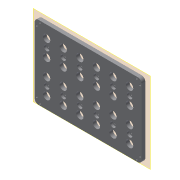
# Autodesk Inventor part: 06_Omniscope_lid_lenses
Saved by Autodesk Inventor 2019 (Build 230136000, 136)
## iProperties
Created: 2021-09-23
Part Number: 06_Omniscope_lid_lenses
Material: Generisch
Document SubType Name: Modeling
Designer: Muriel
Density: 1 g/cm^3
Appearance: Vorgabe
Author: Muriel
Autodesk Inventor part; units mm, degrees
ref_plane "YZ Plane" through (0, 0, 0) normal (1, 0, 0) x (0, 1, 0)
ref_plane "XZ Plane" through (0, 0, 0) normal (0, 1, 0) x (-1, 0, 0)
ref_plane "XY Plane" through (0, 0, 0) normal (0, 0, 1) x (1, 0, 0)
ref_plane "Arbeitsebene1" through (0, 0, 0) normal (0, 0, 1) x (1, 0, 0)
sketch "Skizze1" plane through (0, 0, 0) normal (0, 0, 1) x (1, 0, 0)
  circle A0 centre (-56, 33.5) radius 0.9 projected
  circle A1 centre (-52.5, -38) radius 0.9 projected
  circle A2 centre (56, -33.5) radius 0.9 projected
  circle A3 centre (52.5, 38) radius 0.9 projected
  circle A4 centre (56, 33.5) radius 0.9 projected
  circle A5 centre (52.5, -38) radius 0.9 projected
  circle A6 centre (-56, -33.5) radius 0.9 projected
  circle A7 centre (-52.5, 38) radius 0.9 projected
  line L0 (54.4717, 36.4176) -> (-54.4717, 36.4176) projected
  line L1 (54.4717, -36.4176) -> (54.4717, 36.4176) projected
  line L2 (-54.4717, -36.4176) -> (54.4717, -36.4176) projected
  line L3 (-54.4717, 36.4176) -> (-54.4717, -36.4176) projected
  arc A8 (-57.9717, -35.9176) -> (-53.9717, -39.9176) centre (-53.9717, -35.9176) ccw projected
  line L4 (53.9717, -39.9176) -> (-53.9717, -39.9176) projected
  arc A9 (53.9717, -39.9176) -> (57.9717, -35.9176) centre (53.9717, -35.9176) ccw projected
  line L5 (57.9717, 35.9176) -> (57.9717, -35.9176) projected
  arc A10 (57.9717, 35.9176) -> (53.9717, 39.9176) centre (53.9717, 35.9176) ccw projected
  line L6 (-53.9717, 39.9176) -> (53.9717, 39.9176) projected
  arc A11 (-53.9717, 39.9176) -> (-57.9717, 35.9176) centre (-53.9717, 35.9176) ccw projected
  line L7 (-57.9717, -35.9176) -> (-57.9717, 35.9176) projected
  circle A12 centre (44.9634, -18.0176) radius 1.4 projected
  circle A13 centre (26.9634, -18.0176) radius 1.4 projected
  circle A14 centre (8.9634, -18.0176) radius 1.4 projected
  circle A15 centre (-9.0366, -18.0176) radius 1.4 projected
  circle A16 centre (-27.0366, -18.0176) radius 1.4 projected
  circle A17 centre (-45.0366, -18.0176) radius 1.4 projected
  circle A18 centre (-45.0366, 17.9824) radius 1.4 projected
  circle A19 centre (-27.0366, 17.9824) radius 1.4 projected
  circle A20 centre (-9.0366, 17.9824) radius 1.4 projected
  circle A21 centre (8.9634, 17.9824) radius 1.4 projected
  circle A22 centre (26.9634, 17.9824) radius 1.4 projected
  circle A23 centre (44.9634, 17.9824) radius 1.4 projected
  circle A24 centre (44.9634, -26.9676) radius 4 projected
  circle A25 centre (26.9634, -26.9676) radius 4 projected
  circle A26 centre (8.9634, -26.9676) radius 4 projected
  circle A27 centre (-9.0366, -26.9676) radius 4 projected
  circle A28 centre (-27.0366, -26.9676) radius 4 projected
  circle A29 centre (-45.0366, -26.9676) radius 4 projected
  circle A30 centre (-45.0366, -9.0676) radius 4 projected
  circle A31 centre (-27.0366, -9.0676) radius 4 projected
  circle A32 centre (-9.0366, -9.0676) radius 4 projected
  circle A33 centre (8.9634, -9.0676) radius 4 projected
  circle A34 centre (26.9634, -9.0676) radius 4 projected
  line L8 (47.4634, -11.0176) -> (47.4634, -8.0176) projected
  circle A35 centre (44.9634, -9.0676) radius 4 projected
  circle A36 centre (44.9634, 9.0324) radius 4 projected
  circle A37 centre (44.9634, 26.9324) radius 4 projected
  circle A38 centre (26.9634, 9.0324) radius 4 projected
  circle A39 centre (26.9634, 26.9324) radius 4 projected
  circle A40 centre (8.9634, 9.0324) radius 4 projected
  circle A41 centre (8.9634, 26.9324) radius 4 projected
  circle A42 centre (-9.0366, 26.9324) radius 4 projected
  circle A43 centre (-9.0366, 9.0324) radius 4 projected
  circle A44 centre (-27.0366, 9.0324) radius 4 projected
  circle A45 centre (-27.0366, 26.9324) radius 4.2 projected
  circle A46 centre (-45.0366, 9.0324) radius 4.2 projected
  circle A47 centre (-45.0366, 26.9324) radius 4 projected
  point P0 (0, 0)
extrude "Extrusion1" add sketch "Skizze1" along normal blind 2 contours L1 L2 L3 L0 | L7 A11 L6 A10 L5 A9 L4 A8
sketch "Skizze2" plane through (0, 0, 2) normal (0, 0, 1) x (1, 0, 0)
  circle A0 centre (-45.0366, 9.0324) radius 4.2 projected
  circle A1 centre (-27.0366, 26.9324) radius 4.2 projected
  circle A2 centre (-45.0366, 26.9324) radius 4 projected
  circle A3 centre (-27.0366, 9.0324) radius 4 projected
  circle A4 centre (-9.0366, 9.0324) radius 4 projected
  circle A5 centre (-9.0366, 26.9324) radius 4 projected
  circle A6 centre (8.9634, 26.9324) radius 4 projected
  circle A7 centre (8.9634, 9.0324) radius 4 projected
  circle A8 centre (26.9634, 26.9324) radius 4 projected
  circle A9 centre (26.9634, 9.0324) radius 4 projected
  circle A10 centre (44.9634, 26.9324) radius 4 projected
  circle A11 centre (44.9634, 9.0324) radius 4 projected
  circle A12 centre (44.9634, -9.0676) radius 4 projected
  circle A13 centre (26.9634, -9.0676) radius 4 projected
  circle A14 centre (8.9634, -9.0676) radius 4 projected
  circle A15 centre (-9.0366, -9.0676) radius 4 projected
  circle A16 centre (-27.0366, -9.0676) radius 4 projected
  circle A17 centre (-45.0366, -9.0676) radius 4 projected
  circle A18 centre (-45.0366, -26.9676) radius 4 projected
  circle A19 centre (-27.0366, -26.9676) radius 4 projected
  circle A20 centre (-9.0366, -26.9676) radius 4 projected
  circle A21 centre (8.9634, -26.9676) radius 4 projected
  circle A22 centre (26.9634, -26.9676) radius 4 projected
  circle A23 centre (44.9634, -26.9676) radius 4 projected
  circle A24 centre (44.9634, 17.9824) radius 1.4 projected
  circle A25 centre (26.9634, 17.9824) radius 1.4 projected
  circle A26 centre (8.9634, 17.9824) radius 1.4 projected
  circle A27 centre (-9.0366, 17.9824) radius 1.4 projected
  circle A28 centre (-27.0366, 17.9824) radius 1.4 projected
  circle A29 centre (-45.0366, 17.9824) radius 1.4 projected
  circle A30 centre (-45.0366, -18.0176) radius 1.4 projected
  circle A31 centre (-27.0366, -18.0176) radius 1.4 projected
  circle A32 centre (-9.0366, -18.0176) radius 1.4 projected
  circle A33 centre (8.9634, -18.0176) radius 1.4 projected
  circle A34 centre (26.9634, -18.0176) radius 1.4 projected
  circle A35 centre (44.9634, -18.0176) radius 1.4 projected
  circle A36 centre (-52.5, 38) radius 0.9 projected
  circle A37 centre (-56, -33.5) radius 0.9 projected
  circle A38 centre (52.5, -38) radius 0.9 projected
  circle A39 centre (56, 33.5) radius 0.9 projected
  circle A40 centre (52.5, 38) radius 0.9 projected
  circle A41 centre (56, -33.5) radius 0.9 projected
  circle A42 centre (-52.5, -38) radius 0.9 projected
  circle A43 centre (-56, 33.5) radius 0.9 projected
  arc A44 (-57.9717, -35.9176) -> (-53.9717, -39.9176) centre (-53.9717, -35.9176) ccw projected
  line L0 (-53.9717, -39.9176) -> (53.9717, -39.9176) projected
  arc A45 (53.9717, -39.9176) -> (57.9717, -35.9176) centre (53.9717, -35.9176) ccw projected
  line L1 (57.9717, -35.9176) -> (57.9717, 35.9176) projected
  arc A46 (57.9717, 35.9176) -> (53.9717, 39.9176) centre (53.9717, 35.9176) ccw projected
  line L2 (53.9717, 39.9176) -> (-53.9717, 39.9176) projected
  arc A47 (-53.9717, 39.9176) -> (-57.9717, 35.9176) centre (-53.9717, 35.9176) ccw projected
  line L3 (-57.9717, 35.9176) -> (-57.9717, -35.9176) projected
  point P0 (0, 0)
extrude "Extrusion2" add sketch "Skizze2" along normal blind 2 contours A0 | A1 | A2 | A3 | A4 | A5 | A6 | A7 | A8 | A9 | A10 | A11 | A12 | A13 | A14 | A15 | A16 | A17 | A18 | A19 | A20 | A21 | A22 | A23 | L3 A47 L2 A46 L1 A45 L0 A44
sketch "Skizze3" plane through (0, 0, 4) normal (0, 0, 1) x (1, 0, 0)
  circle A0 centre (44.9634, 17.9824) radius 1.4 projected
  circle A1 centre (48.8634, 17.9824) radius 0.1 projected
  line L0 (52.8634, 35.8824) -> (53.8634, 34.8824) projected
  line L1 (37.0634, 35.8824) -> (52.8634, 35.8824) projected
  line L2 (36.0634, 34.8824) -> (37.0634, 35.8824) projected
  line L3 (36.0634, 1.0824) -> (36.0634, 34.8824) projected
  line L4 (37.0634, 0.0824) -> (36.0634, 1.0824) projected
  line L5 (37.0634, 0.0824) -> (52.8634, 0.0824) projected
  line L6 (53.8634, 1.0824) -> (52.8634, 0.0824) projected
  line L7 (53.8634, 1.0824) -> (53.8634, 34.8824) projected
  circle A2 centre (44.9634, 26.9324) radius 4.2 projected
  circle A3 centre (44.9634, 9.0324) radius 4.2 projected
  circle A4 centre (44.9634, 26.9324) radius 3.95
  circle A5 centre (44.9634, 9.0324) radius 3.95
  point P0 (0, 0)
  dimension "d4" = 7.9
  dimension "d7" = 7.9
  constraints: 2 centre point, 2 coincident
  measures "d4" diameter of A4
  measures "d7" diameter of A5
extrude "Extrusion3" cut sketch "Skizze3" against normal blind 2 contours A4 | A5
sketch "Skizze4" plane through (0, 0, 4) normal (0, 0, 1) x (1, 0, 0)
  circle A0 centre (44.9634, 26.9324) radius 3.95 projected
  circle A1 centre (44.9634, 9.0324) radius 3.95 projected
  circle A2 centre (44.9634, -18.0176) radius 1.4 projected
  circle A3 centre (26.9634, -18.0176) radius 1.4 projected
  circle A4 centre (8.9634, -18.0176) radius 1.4 projected
  circle A5 centre (-9.0366, -18.0176) radius 1.4 projected
  circle A6 centre (-27.0366, -18.0176) radius 1.4 projected
  circle A7 centre (-45.0366, -18.0176) radius 1.4 projected
  circle A8 centre (-45.0366, 17.9824) radius 1.4 projected
  circle A9 centre (-27.0366, 17.9824) radius 1.4 projected
  circle A10 centre (-9.0366, 17.9824) radius 1.4 projected
  circle A11 centre (8.9634, 17.9824) radius 1.4 projected
  circle A12 centre (26.9634, 17.9824) radius 1.4 projected
  circle A13 centre (44.9634, 17.9824) radius 1.4 projected
  circle A14 centre (-56, 33.5) radius 0.9 projected
  circle A15 centre (-52.5, -38) radius 0.9 projected
  circle A16 centre (56, -33.5) radius 0.9 projected
  circle A17 centre (52.5, 38) radius 0.9 projected
  circle A18 centre (56, 33.5) radius 0.9 projected
  circle A19 centre (52.5, -38) radius 0.9 projected
  circle A20 centre (-56, -33.5) radius 0.9 projected
  circle A21 centre (-52.5, 38) radius 0.9 projected
  arc A22 (-57.9717, -35.9176) -> (-53.9717, -39.9176) centre (-53.9717, -35.9176) ccw projected
  line L0 (-53.9717, -39.9176) -> (53.9717, -39.9176) projected
  arc A23 (53.9717, -39.9176) -> (57.9717, -35.9176) centre (53.9717, -35.9176) ccw projected
  line L1 (57.9717, -35.9176) -> (57.9717, 35.9176) projected
  arc A24 (57.9717, 35.9176) -> (53.9717, 39.9176) centre (53.9717, 35.9176) ccw projected
  line L2 (53.9717, 39.9176) -> (-53.9717, 39.9176) projected
  arc A25 (-53.9717, 39.9176) -> (-57.9717, 35.9176) centre (-53.9717, 35.9176) ccw projected
  line L3 (-57.9717, 35.9176) -> (-57.9717, -35.9176) projected
  point P0 (0, 0)
hole "Bohrung1" at (44.9634, -18.0176, 4) at (26.9634, -18.0176, 4) at (8.9634, -18.0176, 4) at (-9.0366, -18.0176, 4) at (-27.0366, -18.0176, 4) at (-45.0366, -18.0176, 4) at (-45.0366, 17.9824, 4) at (-27.0366, 17.9824, 4) at (-9.0366, 17.9824, 4) at (8.9634, 17.9824, 4) at (26.9634, 17.9824, 4) at (44.9634, 17.9824, 4) direction (0, 0, -1) diameter 2.8 depth 12 tip angle 118 counterbore diameter 6 counterbore depth 2.5
pattern_linear "Rechteckige Anordnung1" count 2 spacing 36 along (0, -1, 0) count 6 spacing 18 along (-1, 0, 0) of "Extrusion3"
ref_plane "Arbeitsebene2" through (-53.9717, 0, 0) normal (0, 1, 0) x (1, 0, 0)
ref_plane "Arbeitsebene3" through (0, -35.9176, 0) normal (1, 0, 0) x (0, 0, -1)
sketch "Skizze5" plane through (0, 0, 0) normal (0, 0, -1) x (-1, 0, 0)
  circle A0 centre (56, -33.5) radius 0.9 projected
  circle A1 centre (-56, 33.5) radius 0.9 projected
  circle A2 centre (-56, -33.5) radius 0.9 projected
  circle A3 centre (56, 33.5) radius 0.9 projected
  circle A4 centre (52.5, -38) radius 0.9 projected
  circle A5 centre (-52.5, 38) radius 0.9 projected
  circle A6 centre (-52.5, -38) radius 0.9 projected
  circle A7 centre (52.5, 38) radius 0.9 projected
  arc A8 (53.9717, -39.9176) -> (57.9717, -35.9176) centre (53.9717, -35.9176) ccw projected
  line L0 (57.9717, -35.9176) -> (57.9717, 35.9176) projected
  arc A9 (57.9717, 35.9176) -> (53.9717, 39.9176) centre (53.9717, 35.9176) ccw projected
  line L1 (53.9717, 39.9176) -> (-53.9717, 39.9176) projected
  arc A10 (-53.9717, 39.9176) -> (-57.9717, 35.9176) centre (-53.9717, 35.9176) ccw projected
  line L2 (-57.9717, 35.9176) -> (-57.9717, -35.9176) projected
  arc A11 (-57.9717, -35.9176) -> (-53.9717, -39.9176) centre (-53.9717, -35.9176) ccw projected
  line L3 (-53.9717, -39.9176) -> (53.9717, -39.9176) projected
  circle A12 centre (50.0366, -8.0176) radius 1.4 projected
  circle A13 centre (50.0366, -28.0176) radius 1.4 projected
  circle A14 centre (40.0366, -28.0176) radius 1.4 projected
  circle A15 centre (40.0366, -8.0176) radius 1.4 projected
  circle A16 centre (32.0366, -8.0176) radius 1.4 projected
  circle A17 centre (32.0366, -28.0176) radius 1.4 projected
  circle A18 centre (22.0366, -28.0176) radius 1.4 projected
  circle A19 centre (22.0366, -8.0176) radius 1.4 projected
  circle A20 centre (14.0366, -8.0176) radius 1.4 projected
  circle A21 centre (14.0366, -28.0176) radius 1.4 projected
  circle A22 centre (4.0366, -28.0176) radius 1.4 projected
  circle A23 centre (4.0366, -8.0176) radius 1.4 projected
  circle A24 centre (-3.9634, -8.0176) radius 1.4 projected
  circle A25 centre (-3.9634, -28.0176) radius 1.4 projected
  circle A26 centre (-13.9634, -28.0176) radius 1.4 projected
  circle A27 centre (-13.9634, -8.0176) radius 1.4 projected
  circle A28 centre (-21.9634, -8.0176) radius 1.4 projected
  circle A29 centre (-21.9634, -28.0176) radius 1.4 projected
  circle A30 centre (-31.9634, -28.0176) radius 1.4 projected
  circle A31 centre (-31.9634, -8.0176) radius 1.4 projected
  circle A32 centre (-39.9634, -8.0176) radius 1.4 projected
  circle A33 centre (-39.9634, -28.0176) radius 1.4 projected
  circle A34 centre (-49.9634, -28.0176) radius 1.4 projected
  circle A35 centre (-49.9634, -8.0176) radius 1.4 projected
  circle A36 centre (50.0366, 27.9824) radius 1.4 projected
  circle A37 centre (50.0366, 7.9824) radius 1.4 projected
  circle A38 centre (40.0366, 7.9824) radius 1.4 projected
  circle A39 centre (40.0366, 27.9824) radius 1.4 projected
  circle A40 centre (32.0366, 27.9824) radius 1.4 projected
  circle A41 centre (32.0366, 7.9824) radius 1.4 projected
  circle A42 centre (22.0366, 7.9824) radius 1.4 projected
  circle A43 centre (22.0366, 27.9824) radius 1.4 projected
  circle A44 centre (14.0366, 27.9824) radius 1.4 projected
  circle A45 centre (14.0366, 7.9824) radius 1.4 projected
  circle A46 centre (4.0366, 7.9824) radius 1.4 projected
  circle A47 centre (4.0366, 27.9824) radius 1.4 projected
  circle A48 centre (-3.9634, 27.9824) radius 1.4 projected
  circle A49 centre (-3.9634, 7.9824) radius 1.4 projected
  circle A50 centre (-13.9634, 7.9824) radius 1.4 projected
  circle A51 centre (-13.9634, 27.9824) radius 1.4 projected
  circle A52 centre (-21.9634, 27.9824) radius 1.4 projected
  circle A53 centre (-21.9634, 7.9824) radius 1.4 projected
  circle A54 centre (-31.9634, 7.9824) radius 1.4 projected
  circle A55 centre (-31.9634, 27.9824) radius 1.4 projected
  circle A56 centre (-39.9634, 27.9824) radius 1.4 projected
  circle A57 centre (-39.9634, 7.9824) radius 1.4 projected
  circle A58 centre (-49.9634, 7.9824) radius 1.4 projected
  circle A59 centre (-49.9634, 27.9824) radius 1.4 projected
  arc A60 (-61.6851, 35.0492) -> (-61.8, 34.7718) centre (-59.9, 34.1473) ccw projected
  line L4 (-61.8, -34.7718) -> (-61.8, 34.7718) projected
  arc A61 (-61.8, -34.7718) -> (-61.6851, -35.0492) centre (-59.9, -34.1473) ccw projected
  line L5 (-56.1492, -40.5851) -> (-61.6851, -35.0492) projected
  arc A62 (-56.1492, -40.5851) -> (-55.8718, -40.7) centre (-55.2473, -38.8) ccw projected
  line L6 (60.2, -40.7) -> (-55.8718, -40.7) projected
  arc A63 (60.2, -40.7) -> (61.8, -39.1) centre (60.2, -39.1) ccw projected
  line L7 (61.8, 39.1) -> (61.8, -39.1) projected
  arc A64 (61.8, 39.1) -> (60.2, 40.7) centre (60.2, 39.1) ccw projected
  line L8 (-55.8718, 40.7) -> (60.2, 40.7) projected
  arc A65 (-55.8718, 40.7) -> (-56.1492, 40.5851) centre (-55.2473, 38.8) ccw projected
  line L9 (-61.6851, 35.0492) -> (-56.1492, 40.5851) projected
  line L10 (-54.3, 36.3) -> (54.3, 36.3) projected
  line L11 (54.3, 36.3) -> (54.3, -36.3) projected
  line L12 (54.3, -36.3) -> (-54.3, -36.3) projected
  line L13 (-54.3, -36.3) -> (-54.3, 36.3) projected
  arc A66 (-62.3, -34.8473) -> (-62.092, -35.3494) centre (-59.9, -34.1473) ccw
  line L14 (-62.3, -34.8473) -> (-62.3, 34.8473)
  arc A67 (-62.092, 35.3494) -> (-62.3, 34.8473) centre (-59.9, 34.1473) ccw
  line L15 (-62.092, 35.3494) -> (-56.4494, 40.992)
  arc A68 (-55.9473, 41.2) -> (-56.4494, 40.992) centre (-55.2473, 38.8) ccw
  line L16 (-55.9473, 41.2) -> (60.2, 41.2)
  arc A69 (62.3, 39.1) -> (60.2, 41.2) centre (60.2, 39.1) ccw
  line L17 (62.3, 39.1) -> (62.3, -39.1)
  arc A70 (60.2, -41.2) -> (62.3, -39.1) centre (60.2, -39.1) ccw
  line L18 (60.2, -41.2) -> (-55.9473, -41.2)
  arc A71 (-56.4494, -40.992) -> (-55.9473, -41.2) centre (-55.2473, -38.8) ccw
  line L19 (-56.4494, -40.992) -> (-62.092, -35.3494)
  arc A72 (-61.3, -34.6858) -> (-61.2707, -34.7565) centre (-59.9, -34.1473) ccw
  line L20 (-61.3, -34.6858) -> (-61.3, 34.6858)
  arc A73 (-61.2707, 34.7565) -> (-61.3, 34.6858) centre (-59.9, 34.1473) ccw
  line L21 (-61.2707, 34.7565) -> (-55.8565, 40.1707)
  arc A74 (-55.7858, 40.2) -> (-55.8565, 40.1707) centre (-55.2473, 38.8) ccw
  line L22 (-55.7858, 40.2) -> (60.2, 40.2)
  arc A75 (61.3, 39.1) -> (60.2, 40.2) centre (60.2, 39.1) ccw
  line L23 (61.3, 39.1) -> (61.3, -39.1)
  arc A76 (60.2, -40.2) -> (61.3, -39.1) centre (60.2, -39.1) ccw
  line L24 (60.2, -40.2) -> (-55.7858, -40.2)
  arc A77 (-55.8565, -40.1707) -> (-55.7858, -40.2) centre (-55.2473, -38.8) ccw
  line L25 (-55.8565, -40.1707) -> (-61.2707, -34.7565)
  point P0 (0, 0)
  dimension "d21" = 0.5
  dimension "d22" = 0.5
  constraints: 24 end point, 24 point on circle, 12 centre point, 22 other
  measures "d21" distance between parallel lines of L5 L19
  measures "d22" distance between parallel lines of L5 L25
ref_plane "Arbeitsebene4" through (10.9, -42.3, 2.9) normal (0, 0, -1) x (0, 1, 0)
extrude "Extrusion4" add sketch "Skizze5" against normal up to surface (2.9 mm away) contours L20 A73 L21 A74 L22 A75 L23 A76 L24 A77 L25 A72
